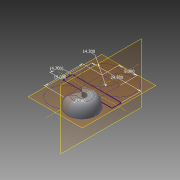
# Autodesk Inventor part: Floor
Saved by Autodesk Inventor 2015 (Build 190159000, 159)
## iProperties
Created: 2016-01-20
Part Number: Floor
Material: Generic
Document SubType Name: Modeling
Designer: sethbattis
Density: 1 g/cm^3
Appearance: Default
Author: sethbattis
Autodesk Inventor part; units mm, degrees
ref_plane "XY Plane" through (0, 0, 0) normal (0, 0, 1) x (1, 0, 0)
sketch "Sketch1" plane through (0, 0, 0) normal (0, 1, 0) x (-1, 0, 0)
  line L0 (311.15, 59.69) -> (-311.15, 59.69)
  line L1 (-311.15, 59.69) -> (-311.15, -59.69)
  line L2 (-311.15, -59.69) -> (311.15, -59.69)
  line L3 (311.15, -59.69) -> (311.15, 59.69)
  line L4 (0, -592.074) -> (0, 592.074) construction
  line L5 (435.61, 0) -> (-435.61, 0) construction
  circle A0 centre (114.3, 241.3) radius 181.61 construction
  circle A1 centre (114.3, -241.3) radius 181.61 construction
  circle A2 centre (-114.3, -241.3) radius 181.61 construction
  line L6 (114.3, 241.3) -> (-114.3, 241.3) construction
  line L7 (114.3, 241.3) -> (114.3, -241.3) construction
  line L8 (114.3, -241.3) -> (-114.3, -241.3) construction
  line L9 (-114.3, -241.3) -> (-114.3, 241.3) construction
  circle A3 centre (-114.3, 241.3) radius 181.61 construction
  line L10 (14.1177, 112.8823) -> (-242.7177, 369.7177) construction
  line L11 (-242.7177, 112.8823) -> (14.1177, 369.7177) construction
  point P0 (0, 0)
  point P1 (-123.7291, 50.5771)
  point P2 (-61.7116, 368.3167)
  point P3 (-114.3, 241.3)
  dimension "d1" = 482.6
  dimension "d3" = 622.3
  dimension "d4" = 119.38
  dimension "d29" = 228.6
  dimension "d30" = 363.22
  dimension "d31" = 45
  constraints: 20 end point, 4 centre point, 4 parallel, 4 point on circle, 3 equal radius, 3 midpoint, 3 perpendicular, 2 tangent, 1 coincident, 1 horizontal, 1 vertical, 3 other
  measures "d1" distance of L6.start L7.end
  measures "d3" distance of L1.end L2.end
  measures "d4" distance of L2.end L0.start
  measures "d29" distance of L7.end L8.end
  measures "d30" diameter of A1
  measures "d31" angle of L6 L10
ref_plane "Work Plane9" through (114.3, 0, -241.3) normal (1, 0, 0) x (0, 0, 1)
sketch "Sketch8" plane through (114.3, 0, -241.3) normal (1, 0, 0) x (0, 0, 1)
  line L0 (354.1823, 0) -> (611.0177, 0) construction
  line L1 (482.6, 0) -> (482.6, -112.6012) construction
  line L2 (482.6, 0) -> (482.6, -57.15)
  line L3 (434.975, -57.15) -> (434.975, -133.35)
  line L4 (434.975, -133.35) -> (374.015, -133.35)
  line L5 (482.6, -57.15) -> (434.975, -57.15)
  line L6 (482.6, 0) -> (300.99, 0)
  ellipse E0 centre (374.015, 0) end of major axis (374.015, -133.35) minor radius 73.025
  point P0 (241.3, 0)
  dimension "d56" = 73.025
  dimension "d52" = 133.35
  dimension "d53" = 181.61
  dimension "d54" = 76.2
  dimension "d55" = 47.625
  constraints: 12 end point, 3 horizontal, 2 point on line, 2 vertical, 1 midpoint, 1 perpendicular, 4 other
  measures "d52" distance between parallel lines of L0 L4
  measures "d53" distance of L1.start L6.end
  measures "d54" distance of L3.start L3.end
  measures "d55" distance of L2.end L3.start
revolve "Revolution2" add sketch "Sketch8" angle 45 about axis through (114.3, 0, 241.3) along (0, 1, 0) and the other way 225 contours L2 L5 E0 L6 | E0 L5 L3 L6 | L3 L4 E0
ref_plane "Work Plane11" through (0, 0, 0) normal (0, 1, 0) x (-1, 0, 0)
sketch "Sketch11" plane through (0, 0, 0) normal (0, 1, 0) x (-1, 0, 0)
  circle A0 centre (-112.9405, 241.9063) radius 127
  point P0 (0, 0)
  dimension "d60" = 254
  constraints: 1 centre point
  measures "d60" diameter of A0
extrude "Extrusion5" add sketch "Sketch11" along normal blind 79.375
body "Solid4"
